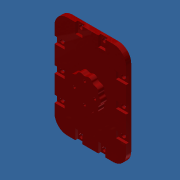
# Autodesk Inventor part: magnetic1-1
Saved by Autodesk Inventor 2015 (Build 190159000, 159)
## iProperties
Created: 2019-02-02
Part Number: magnetic1-1
Material: Generic
Document SubType Name: Modeling
Designer: gabriel
Density: 1 g/cm^3
Appearance: Default
Author: gabriel
Autodesk Inventor part; units mm, degrees
ref_plane "YZ Plane" through (0, 0, 0) normal (1, 0, 0) x (0, 1, 0)
ref_plane "XZ Plane" through (0, 0, 0) normal (0, 1, 0) x (-1, 0, 0)
ref_plane "XY Plane" through (0, 0, 0) normal (0, 0, 1) x (1, 0, 0)
sketch "Sketch27" plane through (0, 0, 0) normal (0, 0, 1) x (1, 0, 0)
  line L0 (0, -7.9375) -> (-28.575, -7.9375)
  line L1 (-36.5125, 0) -> (-36.5125, 47.625)
  line L2 (-28.575, 55.5625) -> (0, 55.5625)
  line L3 (7.9375, 47.625) -> (7.9375, 0)
  circle A0 centre (-28.575, 47.625) radius 6.5484
  circle A1 centre (-28.575, 31.75) radius 6.5484
  circle A2 centre (-28.575, 15.875) radius 6.5484
  circle A3 centre (-28.575, 0) radius 6.5484
  circle A4 centre (-14.2875, 0) radius 6.5484
  circle A5 centre (-14.2875, 47.625) radius 6.5484
  circle A6 centre (0, 47.625) radius 6.5484
  circle A7 centre (0, 31.75) radius 6.5484
  circle A8 centre (0, 15.875) radius 6.5484
  circle A9 centre (0, 0) radius 6.5484
  arc A10 (-28.575, 55.5625) -> (-36.5125, 47.625) centre (-28.575, 47.625) ccw
  arc A11 (7.9375, 47.625) -> (0, 55.5625) centre (0, 47.625) ccw
  arc A12 (-36.5125, 0) -> (-28.575, -7.9375) centre (-28.575, 0) ccw
  arc A13 (0, -7.9375) -> (7.9375, 0) centre (0, 0) ccw
  circle A14 centre (-33.3375, 39.6875) radius 1.3891
  circle A15 centre (-33.3375, 23.8125) radius 1.3891
  circle A16 centre (-33.3375, 7.9375) radius 1.3891
  circle A17 centre (4.7625, 39.6875) radius 1.3891
  circle A18 centre (4.7625, 23.8125) radius 1.3891
  circle A19 centre (4.7625, 7.9375) radius 1.3891
  circle A20 centre (-21.4312, 53.1812) radius 1.3891
  circle A21 centre (-7.1437, 53.1812) radius 1.3891
  circle A22 centre (-21.4312, -5.5562) radius 1.3891
  circle A23 centre (-7.1437, -5.5562) radius 1.3891
  dimension "d126" = 13.0969
  dimension "d127" = 13.0969
  dimension "d128" = 13.0969
  dimension "d129" = 13.0969
  dimension "d130" = 13.0969
  dimension "d131" = 13.0969
  dimension "d132" = 13.0969
  dimension "d133" = 13.0969
  dimension "d134" = 13.0969
  dimension "d135" = 13.0969
  dimension "d136" = 7.9375
  dimension "d137" = 14.2875
  dimension "d138" = 14.2875
  dimension "d139" = 7.9375
  dimension "d140" = 7.9375
  dimension "d141" = 15.875
  dimension "d142" = 15.875
  dimension "d145" = 44.45
  dimension "d146" = 63.5
  dimension "d149" = 2.7781
  dimension "d150" = 2.7781
  dimension "d151" = 2.7781
  dimension "d152" = 2.7781
  dimension "d153" = 2.7781
  dimension "d154" = 2.7781
  dimension "d155" = 3.175
  dimension "d156" = 3.175
  dimension "d157" = 15.875
  dimension "d158" = 15.875
  dimension "d159" = 15.875
  dimension "d162" = 2.7781
  dimension "d163" = 2.7781
  dimension "d164" = 2.7781
  dimension "d165" = 2.7781
  dimension "d166" = 2.3813
  dimension "d169" = 2.3813
  dimension "d170" = 7.1437
  dimension "d171" = 7.1437
  constraints: 24 centre point, 13 vertical alignment, 11 horizontal alignment, 8 end point, 8 point on circle, 5 coincident, 4 tangent, 2 parallel, 1 horizontal, 1 perpendicular
  measures "d126" diameter of A0
  measures "d127" diameter of A1
  measures "d128" diameter of A2
  measures "d129" diameter of A3
  measures "d130" diameter of A4
  measures "d131" diameter of A9
  measures "d132" diameter of A8
  measures "d133" diameter of A7
  measures "d134" diameter of A6
  measures "d135" diameter of A5
  measures "d136" distance from line of L1 A0.centre
  measures "d137" distance of A5.centre A0.centre
  measures "d138" distance of A5.centre A6.centre
  measures "d139" distance from line of L2 A0.centre
  measures "d140" distance from line of L0 A3.centre
  measures "d141" distance of A2.centre A3.centre
  measures "d142" distance of A0.centre A1.centre
  measures "d145" distance between parallel lines of L3 L1
  measures "d146" distance between parallel lines of L0 L2
  measures "d149" diameter of A14
  measures "d150" diameter of A15
  measures "d151" diameter of A16
  measures "d152" diameter of A17
  measures "d153" diameter of A18
  measures "d154" diameter of A19
  measures "d155" distance from line of L1 A14.centre
  measures "d156" distance from line of L3 A17.centre
  measures "d157" distance from line of L2 A14.centre
  measures "d158" distance of A15.centre A14.centre
  measures "d159" distance of A15.centre A16.centre
  measures "d162" diameter of A20
  measures "d163" diameter of A21
  measures "d164" diameter of A22
  measures "d165" diameter of A23
  measures "d166" distance from line of L2 A20.centre
  measures "d169" distance from line of L0 A22.centre
  measures "d170" horizontal distance of A10.centre A20.centre
  measures "d171" horizontal distance of A21.centre A5.centre
extrude "Extrusion25" add sketch "Sketch27" along normal blind 3.175 contours L0 A12 L1 A10 L2 A11 L3 A13 | A0 | A1 | A2 | A3 | A4 | A5 | A6 | A7 | A8 | A9
sketch "Sketch38" plane through (0, 0, 3.175) normal (0, 0, 1) x (1, 0, 0)
  circle A0 centre (-14.2875, 23.8125) radius 9.525
  arc A1 (-15.4885, 33.2615) -> (-18.8698, 32.1628) centre (-16.6896, 31.2053) ccw
  arc A2 (-15.4885, 33.2615) -> (-13.0865, 33.2615) centre (-14.2875, 35.3177) ccw
  line L0 (7.9375, 0) -> (7.9375, 47.625) projected
  line L1 (0, 55.5625) -> (-28.575, 55.5625) projected
  arc A3 (-9.7052, 32.1628) -> (-13.0865, 33.2615) centre (-11.8854, 31.2053) ccw
  arc A4 (-9.7052, 32.1628) -> (-7.7619, 30.7509) centre (-7.5249, 33.1204) ccw
  arc A5 (-5.6721, 27.8746) -> (-7.7619, 30.7509) centre (-7.9988, 28.3815) ccw
  arc A6 (-5.6721, 27.8746) -> (-4.9299, 25.5901) centre (-3.3454, 27.3678) ccw
  arc A7 (-4.9299, 22.0349) -> (-4.9299, 25.5901) centre (-6.5143, 23.8125) ccw
  arc A8 (-4.9299, 22.0349) -> (-5.6721, 19.7504) centre (-3.3454, 20.2572) ccw
  arc A9 (-7.7619, 16.8741) -> (-5.6721, 19.7504) centre (-7.9988, 19.2435) ccw
  arc A10 (-7.7619, 16.8741) -> (-9.7052, 15.4622) centre (-7.5249, 14.5046) ccw
  arc A11 (-13.0865, 14.3635) -> (-9.7052, 15.4622) centre (-11.8854, 16.4197) ccw
  arc A12 (-13.0865, 14.3635) -> (-15.4885, 14.3635) centre (-14.2875, 12.3073) ccw
  arc A13 (-18.8698, 15.4622) -> (-15.4885, 14.3635) centre (-16.6896, 16.4197) ccw
  arc A14 (-18.8698, 15.4622) -> (-20.8131, 16.8741) centre (-21.0501, 14.5046) ccw
  arc A15 (-22.9029, 19.7504) -> (-20.8131, 16.8741) centre (-20.5762, 19.2435) ccw
  arc A16 (-22.9029, 19.7504) -> (-23.6451, 22.0349) centre (-25.2296, 20.2572) ccw
  arc A17 (-20.8131, 30.7509) -> (-18.8698, 32.1628) centre (-21.0501, 33.1204) ccw
  arc A18 (-23.6451, 25.5901) -> (-23.6451, 22.0349) centre (-22.0607, 23.8125) ccw
  arc A19 (-23.6451, 25.5901) -> (-22.9029, 27.8746) centre (-25.2296, 27.3678) ccw
  arc A20 (-20.8131, 30.7509) -> (-22.9029, 27.8746) centre (-20.5762, 28.3815) ccw
  point P0 (0, 0)
  dimension "d265" = 19.05
  dimension "d266" = 22.225
  dimension "d267" = 31.75
  dimension "d268" = 2.3813
  constraints: 40 point on circle, 38 equal radius, 20 centre point, 1 vertical alignment, 22 other
  measures "d266" distance from line of L0 point (-14.288, 23.812)
  measures "d267" distance from line of L1 point (-14.288, 23.812)
  measures "d268" radius of A1
extrude "Extrusion29" add sketch "Sketch38" along normal blind 3.5719 contours A0 A8 A10 A12 A14 A16 A19 A17 A2 A4 A6 | A0 A7 | A0 A5 | A9 A0 | A0 A3 | A11 A0 | A0 A1 | A13 A0 | A0 A20 | A15 A0 | A0 A18
sketch "Sketch39" plane through (0, 0, 3.175) normal (0, 0, 1) x (1, 0, 0)
  line L0 (7.9375, 10.1203) -> (1.5875, 10.1203)
  line L1 (1.5875, 10.1203) -> (1.5875, 5.7547)
  line L2 (1.5875, 5.7547) -> (7.9375, 5.7547)
  line L3 (7.9375, 5.7547) -> (7.9375, 10.1203)
  line L4 (7.9375, 0) -> (7.9375, 47.625) projected
  circle A0 centre (4.7625, 7.9375) radius 1.3891 projected
  line L5 (7.9375, 25.9953) -> (1.5875, 25.9953)
  line L6 (1.5875, 25.9953) -> (1.5875, 21.6297)
  line L7 (1.5875, 21.6297) -> (7.9375, 21.6297)
  line L8 (7.9375, 21.6297) -> (7.9375, 25.9953)
  line L9 (7.9375, 41.8703) -> (1.5875, 41.8703)
  line L10 (1.5875, 41.8703) -> (1.5875, 37.5047)
  line L11 (1.5875, 37.5047) -> (7.9375, 37.5047)
  line L12 (7.9375, 37.5047) -> (7.9375, 41.8703)
  line L13 (0, 55.5625) -> (-28.575, 55.5625) projected
  line L14 (-9.3266, 55.5625) -> (-4.9609, 55.5625)
  line L15 (-4.9609, 55.5625) -> (-4.9609, 49.2125)
  line L16 (-4.9609, 49.2125) -> (-9.3266, 49.2125)
  line L17 (-9.3266, 49.2125) -> (-9.3266, 55.5625)
  line L18 (-19.2484, 55.5625) -> (-23.6141, 55.5625)
  line L19 (-23.6141, 55.5625) -> (-23.6141, 49.2125)
  line L20 (-23.6141, 49.2125) -> (-19.2484, 49.2125)
  line L21 (-19.2484, 49.2125) -> (-19.2484, 55.5625)
  line L22 (-36.5125, 41.8703) -> (-30.1625, 41.8703)
  line L23 (-30.1625, 41.8703) -> (-30.1625, 37.5047)
  line L24 (-30.1625, 37.5047) -> (-36.5125, 37.5047)
  line L25 (-36.5125, 37.5047) -> (-36.5125, 41.8703)
  line L26 (-36.5125, 25.9953) -> (-30.1625, 25.9953)
  line L27 (-30.1625, 25.9953) -> (-30.1625, 21.6297)
  line L28 (-30.1625, 21.6297) -> (-36.5125, 21.6297)
  line L29 (-36.5125, 21.6297) -> (-36.5125, 25.9953)
  line L30 (-36.5125, 10.1203) -> (-30.1625, 10.1203)
  line L31 (-30.1625, 10.1203) -> (-30.1625, 5.7547)
  line L32 (-30.1625, 5.7547) -> (-36.5125, 5.7547)
  line L33 (-36.5125, 5.7547) -> (-36.5125, 10.1203)
  line L34 (0, -7.9375) -> (-28.575, -7.9375) projected
  line L35 (-23.6141, -7.9375) -> (-19.2484, -7.9375)
  line L36 (-19.2484, -7.9375) -> (-19.2484, -1.5875)
  line L37 (-19.2484, -1.5875) -> (-23.6141, -1.5875)
  line L38 (-23.6141, -1.5875) -> (-23.6141, -7.9375)
  line L39 (-9.3266, -7.9375) -> (-4.9609, -7.9375)
  line L40 (-4.9609, -7.9375) -> (-4.9609, -1.5875)
  line L41 (-4.9609, -1.5875) -> (-9.3266, -1.5875)
  line L42 (-9.3266, -1.5875) -> (-9.3266, -7.9375)
  line L43 (-36.5125, 47.625) -> (-36.5125, 0) projected
  circle A1 centre (4.7625, 23.8125) radius 1.3891 projected
  circle A2 centre (4.7625, 39.6875) radius 1.3891 projected
  circle A3 centre (-7.1437, 53.1812) radius 1.3891 projected
  circle A4 centre (-21.4312, 53.1812) radius 1.3891 projected
  point P0 (0, 0)
  dimension "d273" = 4.3656
  dimension "d274" = 6.35
  dimension "d275" = 2.1828
  dimension "d276" = 2.1828
  dimension "d277" = 2.1828
  dimension "d278" = 2.1828
  dimension "d279" = 2.1828
  constraints: 80 end point, 20 parallel, 15 equal length, 15 point on line, 10 horizontal, 10 perpendicular, 3 collinear
  measures "d273" distance of L0.end L1.end
  measures "d274" distance of L1.end L2.end
  measures "d275" distance from line of A0.centre L0
  measures "d276" distance from line of A1.centre L5
  measures "d277" distance from line of A2.centre L9
  measures "d278" distance from line of A3.centre L15
  measures "d279" distance from line of A4.centre L21
extrude "Extrusion30" cut sketch "Sketch39" against normal blind 1.5875
sketch "Sketch41" plane through (0, 0, 6.7469) normal (0, 0, 1) x (1, 0, 0)
  circle A0 centre (-14.2875, 30.1625) radius 0.7937
  circle A1 centre (-14.2875, 17.4625) radius 0.7937
  circle A2 centre (-7.9375, 23.8125) radius 0.7937
  circle A3 centre (-20.6375, 23.8125) radius 0.7937
  line L0 (-9.3266, 55.5625) -> (-19.2484, 55.5625) projected
  line L1 (7.9375, 25.9953) -> (7.9375, 37.5047) projected
  point P0 (0, 0)
  dimension "d287" = 1.5875
  dimension "d288" = 1.5875
  dimension "d289" = 1.5875
  dimension "d290" = 1.5875
  dimension "d291" = 12.7
  dimension "d292" = 12.7
  dimension "d293" = 6.35
  dimension "d294" = 6.35
  dimension "d295" = 25.4
  dimension "d296" = 15.875
  constraints: 4 centre point, 1 horizontal alignment, 1 vertical alignment
  measures "d287" diameter of A1
  measures "d288" diameter of A2
  measures "d289" diameter of A0
  measures "d290" diameter of A3
  measures "d291" distance of A2.centre A3.centre
  measures "d292" distance of A1.centre A0.centre
  measures "d293" horizontal distance of A3.centre A0.centre
  measures "d294" horizontal distance of A1.centre A3.centre
  measures "d295" distance from line of L0 A0.centre
  measures "d296" distance from line of L1 A2.centre
extrude "Extrusion32" cut sketch "Sketch41" against normal through all
equation "\"d127\" = d126"
equation "\"d128\" = d126"
equation "\"d129\" = d126"
equation "\"d130\" = d126"
equation "\"d131\" = d126"
equation "\"d132\" = d126"
equation "\"d133\" = d126"
equation "\"d134\" = d126"
equation "\"d135\" = d126"
equation "\"d138\" = d137"
equation "\"d139\" = d136"
equation "\"d140\" = d136"
equation "\"d142\" = d141"
equation "\"d150\" = d149"
equation "\"d151\" = d149"
equation "\"d152\" = d149"
equation "\"d153\" = d149"
equation "\"d154\" = d149"
equation "\"d158\" = d157"
equation "\"d159\" = d157"
equation "\"d162\" = d149"
equation "\"d163\" = d149"
equation "\"d164\" = d149"
equation "\"d165\" = d149"
equation "\"d170\" = 0.5 * d137"
equation "\"d171\" = d170"
body "Solid9"
